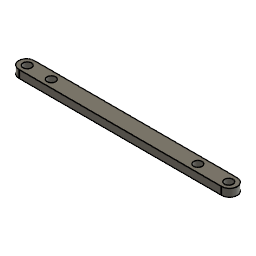
barra_soportes_giratorios_v3 (Autodesk Fusion 360 design; units mm, degrees)
part number: 2026-03-18-00-43-48-154
Autodesk Fusion 360 part; units mm, degrees
sketch "Boceto1" plane through (0, 0, 0) normal (0, 1, 0) x (1, 0, 0)
  line L0 (-63, -5) -> (67.4, -5)
  line L1 (67.4, 5) -> (-63, 5)
  line L2 (-67.4, 0) -> (67.4, 0) construction
  circle A0 centre (67.4, 0) radius 2.75
  circle A1 centre (-63, 0) radius 2.75
  arc A2 (-63, 5) -> (-63.25, 4.9937) centre (-63, 0) ccw
  arc A3 (-63.25, -4.9937) -> (-63, -5) centre (-63, 0) ccw
  arc A4 (-63.25, 4.9937) -> (-63.25, -4.9937) centre (-63.5, 0) ccw
  arc A5 (67.4, -5) -> (67.65, -4.9937) centre (67.4, 0) ccw
  arc A6 (67.65, 4.9937) -> (67.4, 5) centre (67.4, 0) ccw
  arc A7 (67.65, -4.9937) -> (67.65, 4.9937) centre (67.9, 0) ccw
  dimension "d1" = 10
  dimension "d4" = 5.5
  dimension "d11" = 5.5
  dimension "d12" = 130.4
  dimension "d13" = 10
  dimension "d14" = 0.5
  dimension "d15" = 10
  dimension "d16" = 0.5
  constraint tangent L0 A5
  constraint tangent L1 A6
  constraint parallel L0 L1
  constraint horizontal L2
  constraint midpoint L2 origin
  constraint concentric A0 A5
  constraint coincident L2 A1.centre
  constraint concentric A1 A2
  constraint tangent L1 A2
  constraint coincident L2 A4.centre
  constraint concentric A2 A3
  constraint concentric A5 A6
  measures "d1" distance of L0 L1
  measures "d4" diameter of A0
  measures "d11" diameter of A1
  measures "d12" distance of L2.end A1.centre
  measures "d13" diameter of A4
  measures "d14" distance of A1.centre A4.centre
  measures "d15" diameter of A7
  measures "d16" distance of L2.end A7.centre
extrude "Extruir1" add sketch "Boceto1" along normal blind 5
sketch "Boceto2" plane through (0, 5, 0) normal (0, 1, 0) x (-1, 0, 0)
  circle A0 centre (-67.4, 0) radius 2.75
  line L0 (63, 5) -> (-67.4, 5)
  arc A1 (-67.65, -4.9937) -> (-67.4, -5) centre (-67.4, 0) ccw
  line L1 (-67.4, -5) -> (63, -5)
  circle A2 centre (47.4, 0) radius 2.75
  line L2 (0, 0) -> (0, -16) construction
  circle A3 centre (-47.4, 0) radius 2.75
  arc A4 (-67.65, 4.9937) -> (-67.65, -4.9937) centre (-67.9, 0) ccw
  arc A5 (63, -5) -> (63.25, -4.9937) centre (63, 0) ccw
  arc A6 (63.25, -4.9937) -> (63.25, 4.9937) centre (63.5, 0) ccw
  arc A7 (63.25, 4.9937) -> (63, 5) centre (63, 0) ccw
  arc A8 (-67.4, 5) -> (-67.65, 4.9937) centre (-67.4, 0) ccw
  circle A9 centre (63, 0) radius 2.75
  dimension "d7" = 5.5
  dimension "d17" = 47.4
  dimension "d18" = 47.4
  constraint coincident L2.start origin
  constraint vertical L2
  constraint symmetric A2 L2 A3
  measures "d7" diameter of A2
  measures "d17" distance of L2 A3.centre
  measures "d18" distance of A2.centre L2
extrude "Extruir2" cut sketch "Boceto2" against normal blind 13 contours A2 | A3
